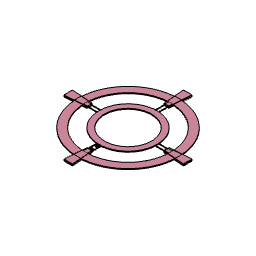
セリカ_ヘイロー_mk1 v2 (Autodesk Fusion 360 design; units mm, degrees)
Autodesk Fusion 360 part; units mm, degrees
sketch "スケッチ1" plane through (0, 0, 0) normal (0, 0, 1) x (1, 0, 0)
sketch "スケッチ1 (2)" plane through (0, 0, 0) normal (0, 0, 1) x (1, 0, 0) in component "Component'"
  circle A0 centre (0, 0) radius 55
  circle A1 centre (0, 0) radius 68
  circle A2 centre (0, 0) radius 100
  circle A3 centre (0, 0) radius 118
  line L0 (-99.92, 4) -> (-67.8823, 4)
  line L1 (-99.92, -4) -> (-67.8823, -4)
  line L2 (0, 0) -> (-118, 0) construction
  line L3 (99.92, -4) -> (67.8823, -4)
  line L4 (99.92, 4) -> (67.8823, 4)
  line L5 (4, 99.92) -> (4, 67.8823)
  line L6 (-4, 99.92) -> (-4, 67.8823)
  line L7 (0, 0) -> (0, -118) construction
  line L8 (-5, -67.8159) -> (-5, -99.8749)
  line L9 (5, -67.8159) -> (5, -99.8749)
  circle A4 centre (0, -73) radius 2.6
  circle A5 centre (0, -85) radius 2.6
  dimension "d9" = 110
  dimension "d10" = 136
  dimension "d11" = 200
  dimension "d12" = 236
  dimension "d13" = 4
  dimension "d15" = 360
  dimension "d37" = 10
  dimension "d38" = 5.2
  dimension "d39" = 5.2
  dimension "d40" = 12
  dimension "d41" = 73
  constraint coincident A0.centre A1.centre
  constraint concentric A0 A1
  constraint concentric A0 A2
  constraint concentric A0 A3
  constraint horizontal L0
  constraint parallel L0 L1
  constraint coincident A3 L2.end
  constraint horizontal L2
  constraint symmetric L0 L1 L2
  constraint coincident A1 L0.end
  constraint coincident A1 L1.end
  constraint coincident A2 L1.start
  constraint coincident A2 L0.start
  constraint coincident A3 L7.end
  constraint perpendicular L2 L7
  constraint coincident A1 L8.start
  constraint coincident A2 L8.end
  constraint vertical L8
  constraint coincident A1 L9.start
  constraint coincident A2 L9.end
  constraint parallel L7 L9
  constraint symmetric L7 L8 L9
  constraint coincident L7 A4.centre
  constraint coincident L7 A5.centre
  measures "d9" diameter of A0
  measures "d10" diameter of A1
  measures "d11" diameter of A2
  measures "d12" diameter of A3
  measures "d13" distance of L0 L2
  measures "d37" distance of L8 L9
  measures "d38" diameter of A4
  measures "d39" diameter of A5
  measures "d40" distance of A4.centre A5.centre
  measures "d41" distance of A0.centre A4.centre
extrude "押し出し1" add sketch "スケッチ1 (2)" along normal blind 2 contours A1 | A3 makes body 1 at (-104.8764, -38.485, 0) makes body 2 at (-59.6004, -21.9197, 2) in component "Component'"
extrude "押し出し2" add sketch "スケッチ1 (2)" along normal blind 2 separate body contours A1 A2 L3 L4 | A1 A2 L5 L6 | A1 A2 L8 L9 | A1 A2 L0 L1 makes body 3 at (-3.1113, 78.5964, 0) makes body 4 at (-78.5964, -3.1113, 0) makes body 5 at (78.5964, -3.1113, 0) makes body 6 at (-0.0648, -95.855, 0) in component "Component'"
sketch "スケッチ1 (3)" plane through (0, 0, 0) normal (0, 0, 1) x (1, 0, 0) in component "Component''"
  line L0 (-140, 7.5) -> (-140, -7.5)
  line L1 (-90, 6) -> (-90, -6)
  line L2 (0, 0) -> (-162.8545, 0) construction
  arc A0 (-99.3711, 5.0623) -> (-99.2713, -6.7417) centre (0, 0) ccw
  arc A1 (-118.212, 8.257) -> (-118.212, -8.257) centre (0, 0) ccw
  line L3 (-90, 4.5) -> (-99.3982, 4.5)
  line L4 (-90, -4.5) -> (-99.3982, -4.5)
  line L5 (-90, -6) -> (-140, -10)
  line L6 (-140, -10) -> (-140, -7.5)
  line L7 (-90, 6) -> (-140, 10)
  line L8 (-140, 10) -> (-140, 7.5)
  arc A2 (-99.2713, 6.7417) -> (-99.3711, 5.0623) centre (0, 0) ccw
  dimension "d22" = 90
  dimension "d23" = 99.5
  dimension "d24" = 118.5
  constraint parallel L0 L1
  constraint coincident L2.start A0.centre
  constraint horizontal L2
  constraint vertical L0
  constraint coincident L1 L3.start
  constraint coincident A0 L3.end
  constraint perpendicular L1 L3
  constraint coincident L1 L4.start
  constraint coincident A0 L4.end
  constraint perpendicular L1 L4
  constraint coincident L7 A2.start
  constraint coincident L5 A0.end
  constraint coincident L5 A1.end
  constraint coincident L7 A1.start
  measures "d22" distance of L2.start L1
  measures "d23" radius of A0
  measures "d24" radius of A1
extrude "押し出し3" add sketch "スケッチ1 (3)" along normal blind 1 separate body makes body 7 in component "Component''"
extrude "押し出し4" add sketch "スケッチ1 (3)" against normal blind 1.2 contours L0 A1 L5 L6 L7 L8 | L1 A0 L3 L7 A2 | L1 A0 L4 L5 bodies 7 in component "Component''"
copy_body "ボディのコピーと貼り付け2" bodies 7 makes body 8 in component "Component''"
move_body "移動4" bodies 8 to x (1, 0, 0) y (0, -1, 0) z (0, 0, -1) at (0, -20, -32.4) in component "Component''"
move_body "移動5" bodies 8 to x (1, 0, 0) y (0, 1, 0) z (0, 0, 1) at (0, 20, 30) in component "Component''"
component_pattern "component pattern"
component "Component'" placed x (1, 0, 0) y (0, 1, 0) z (0, 0, 1) at (0, 0, 0)
component "Component''" placed x (1, 0, 0) y (0, 1, 0) z (0, 0, 1) at (0, 0, 2.2)
component "Component''" placed x (0, 1, 0) y (-1, 0, 0) z (0, 0, 1) at (0, 0, 2.2)
component "Component''" placed x (-1, 0, 0) y (0, -1, 0) z (0, 0, 1) at (0, 0, 2.2)
component "Component''" placed x (0, -1, 0) y (1, 0, 0) z (0, 0, 1) at (0, 0, 2.2)
